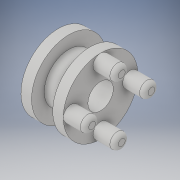
# Autodesk Inventor part: SpoolWindDriver
Saved by Autodesk Inventor 2019 (Build 230136000, 136)
## iProperties
Created: 2019-01-14
Part Number: SpoolWindDriver
Material: Generic
Document SubType Name: Modeling
Designer: Kepler
Density: 1 g/cm^3
Appearance: Default
Author: Kepler
Autodesk Inventor part; units mm, degrees
ref_plane "YZ Plane" through (0, 0, 0) normal (1, 0, 0) x (0, 1, 0)
ref_plane "XZ Plane" through (0, 0, 0) normal (0, 1, 0) x (-1, 0, 0)
ref_plane "XY Plane" through (0, 0, 0) normal (0, 0, 1) x (1, 0, 0)
sketch "Sketch3" plane through (0, 0, 0) normal (0, 0, 1) x (1, 0, 0)
  line L0 (0, 0) -> (0, 5.8)
  line L1 (0, 8.8) -> (10, 8.8)
  line L2 (10, 5.8) -> (10, 0)
  line L3 (10, 0) -> (7.5, 0)
  line L4 (7.5, 0) -> (7.5, 3)
  line L5 (7.5, 3) -> (2.5, 3)
  line L6 (2.5, 3) -> (2.5, 0)
  line L7 (2.5, 0) -> (0, 0)
  line L8 (0, 5.8) -> (10, 5.8)
  dimension "d10" = 8.8
  dimension "d11" = 10
  dimension "d12" = 2.5
  dimension "d13" = 3
  dimension "d14" = 5
  dimension "d24" = 6
  dimension "d25" = 5.8
  constraints: 18 end point, 6 perpendicular, 1 horizontal, 1 parallel, 1 point on line, 1 vertical
  measures "d10" distance of L0.start L1.start
  measures "d11" distance of L1.start L1.end
  measures "d12" distance of L2.end L3.end
  measures "d13" distance of L3.end L4.end
  measures "d14" distance of L4.end L5.end
  measures "d24" diameter of L8 L1
  measures "d25" distance between parallel lines of L3 L8
sketch "Sketch4" plane through (0, 0, 0) normal (0, 0, 1) x (1, 0, 0)
  point P0 (0, 0)
revolve "Revolution1" add sketch "Sketch3" angle 360 about axis through (0, 8.8, 0) along (1, 0, 0)
sketch "Sketch7" plane through (10, 8.8, 0) normal (1, 0, 0) x (0, 0, -1)
  circle A0 centre (7, 0) radius 1.8
  circle A1 centre (-7, 0) radius 1.8
  circle A2 centre (0, -7) radius 1.8
  circle A3 centre (0, 0) radius 8.8 projected
  circle A4 centre (0, 7) radius 1.8
  point P0 (0, -8.8)
  dimension "d27" = 3.6
  dimension "d28" = 3.6
  dimension "d29" = 3.6
  dimension "d30" = 3.6
  constraints: 4 centre point, 1 vertical alignment, 4 other
  measures "d27" diameter of A0
  measures "d28" diameter of A1
  measures "d29" diameter of A2
  measures "d30" diameter of A4
extrude "Extrusion4" add sketch "Sketch7" along normal blind 5 contours A0 | A4 | A1 | A2
fillet "Fillet1" radius 1 1 edges at (15, 15.8, 1.8)
fillet "Fillet2" radius 1 1 edges at (15, 8.8, -5.2)
fillet "Fillet3" radius 1 1 edges at (15, 1.8, 1.8)
fillet "Fillet4" radius 1 1 edges at (15, 8.8, 8.8)
equation "\"d25\" = d10 - 0.5 * d24"
body "Solid2"
